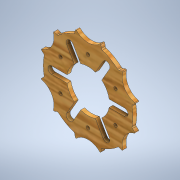
# Autodesk Inventor part: GenevaHolder
Saved by Autodesk Inventor 2020.1 (Build 241239000, 239)
## iProperties
Created: 2019-11-06
Part Number: GenevaHolder
Material: Plywood, Finish
Document SubType Name: Modeling
Designer: Paul Lefeuvre
Density: 0.552 g/cm^3
Appearance: Plywood - New
Author: Paul Lefeuvre
Autodesk Inventor part; units mm, degrees
ref_plane "YZ Plane" through (0, 0, 0) normal (1, 0, 0) x (0, 1, 0)
ref_plane "XZ Plane" through (0, 0, 0) normal (0, 1, 0) x (-1, 0, 0)
ref_plane "XY Plane" through (0, 0, 0) normal (0, 0, 1) x (1, 0, 0)
sketch "Sketch1" plane through (0, 0, 0) normal (0, 0, 1) x (1, 0, 0)
  circle A0 centre (0, 0) radius 175
  circle A1 centre (0, 136.9) radius 38.1
  line L0 (0, 0) -> (0, 152.9684) construction
  circle A2 centre (0, 0) radius 50
  line L1 (0, 0) -> (-42.671, 73.9083)
  line L2 (-31.9973, 38.421) -> (-50.0322, 69.6583)
  line L3 (-17.2749, 46.921) -> (-35.3098, 78.1583)
  arc A3 (-35.3098, 78.1583) -> (-50.0322, 69.6583) centre (-42.671, 73.9083) ccw
  line L4 (-16.7016, 47.1281) -> (-34.7901, 78.4583)
  arc A4 (-34.7901, 78.4583) -> (-50.5518, 69.3583) centre (-42.671, 73.9083) ccw
  line L5 (-50.5518, 69.3583) -> (-32.4633, 38.0281)
  line L6 (-49.1649, 9.1) -> (-85.342, 9.1)
  arc A5 (-85.342, 9.1) -> (-85.342, -9.1) centre (-85.342, 0) ccw
  line L7 (-85.342, -9.1) -> (-49.1649, -9.1)
  line L8 (-49.2722, 8.5) -> (-85.342, 8.5)
  arc A6 (-85.342, 8.5) -> (-85.342, -8.5) centre (-85.342, 0) ccw
  line L9 (-49.2722, -8.5) -> (-85.342, -8.5)
  line L10 (-32.4633, -38.0281) -> (-50.5518, -69.3583)
  arc A7 (-50.5518, -69.3583) -> (-34.7901, -78.4583) centre (-42.671, -73.9083) ccw
  line L11 (-34.7901, -78.4583) -> (-16.7016, -47.1281)
  line L12 (-31.9973, -38.421) -> (-50.0322, -69.6583)
  arc A8 (-50.0322, -69.6583) -> (-35.3098, -78.1583) centre (-42.671, -73.9083) ccw
  line L13 (-17.2749, -46.921) -> (-35.3098, -78.1583)
  line L14 (16.7016, -47.1281) -> (34.7901, -78.4583)
  arc A9 (34.7901, -78.4583) -> (50.5518, -69.3583) centre (42.671, -73.9083) ccw
  line L15 (50.5518, -69.3583) -> (32.4633, -38.0281)
  line L16 (17.2749, -46.921) -> (35.3098, -78.1583)
  arc A10 (35.3098, -78.1583) -> (50.0322, -69.6583) centre (42.671, -73.9083) ccw
  line L17 (31.9973, -38.421) -> (50.0322, -69.6583)
  line L18 (49.1649, -9.1) -> (85.342, -9.1)
  arc A11 (85.342, -9.1) -> (85.342, 9.1) centre (85.342, 0) ccw
  line L19 (85.342, 9.1) -> (49.1649, 9.1)
  line L20 (49.2722, -8.5) -> (85.342, -8.5)
  arc A12 (85.342, -8.5) -> (85.342, 8.5) centre (85.342, 0) ccw
  line L21 (49.2722, 8.5) -> (85.342, 8.5)
  line L22 (32.4633, 38.0281) -> (50.5518, 69.3583)
  arc A13 (50.5518, 69.3583) -> (34.7901, 78.4583) centre (42.671, 73.9083) ccw
  line L23 (34.7901, 78.4583) -> (16.7016, 47.1281)
  line L24 (31.9973, 38.421) -> (50.0322, 69.6583)
  arc A14 (50.0322, 69.6583) -> (35.3098, 78.1583) centre (42.671, 73.9083) ccw
  line L25 (17.2749, 46.921) -> (35.3098, 78.1583)
  arc A15 (49.2722, -8.5) -> (17.2749, 46.921) centre (49.2722, 28.4473) ccw construction
  circle A16 centre (0, 0) radius 93.842 construction
  arc A17 (17.2749, 46.921) -> (49.2722, -8.5) centre (49.2722, 28.4473) ccw construction
  circle A18 centre (49.2722, 28.4473) radius 19.9473 construction
  arc A19 (30.6615, 93.9218) -> (28.3532, 111.45) centre (0, 98.8) ccw
  arc A20 (-28.3532, 111.45) -> (-30.6615, 93.9218) centre (0, 98.8) ccw
  circle A21 centre (0, 0) radius 115 construction
  arc A22 (31.6229, 93.6025) -> (30.2963, 109.2477) centre (0, 98.8) ccw
  arc A23 (-30.2963, 109.2477) -> (-31.6229, 93.6025) centre (0, 98.8) ccw
  arc A24 (-26.9888, 110.0074) -> (26.9888, 110.0074) centre (0, 136.9) ccw
  arc A25 (-26.9888, 110.0074) -> (-30.2963, 109.2477) centre (-28.4056, 108.5957) ccw
  arc A26 (30.2963, 109.2477) -> (26.9888, 110.0074) centre (28.4056, 108.5957) ccw
  arc A27 (31.2727, 102.1077) -> (29.7291, 109.0521) centre (0, 98.8) ccw
  arc A28 (29.7291, 109.0521) -> (27.4139, 109.5839) centre (28.4056, 108.5957) ccw
  arc A29 (-27.4139, 109.5839) -> (27.4139, 109.5839) centre (0, 136.9) ccw
  arc A30 (-27.4139, 109.5839) -> (-29.7291, 109.0521) centre (-28.4056, 108.5957) ccw
  arc A31 (-29.7291, 109.0521) -> (-31.2727, 102.1077) centre (0, 98.8) ccw
  arc A32 (102.8895, -20.9465) -> (102.8895, 20.9465) centre (0, 0) ccw
  arc A33 (-102.8895, 20.9465) -> (-102.8895, -20.9465) centre (0, 0) ccw
  arc A34 (-69.5849, -78.6317) -> (-33.3045, -99.5781) centre (0, 0) ccw
  arc A35 (33.3045, -99.5781) -> (69.5849, -78.6317) centre (0, 0) ccw
  arc A36 (-18.1758, 103.4149) -> (-19.1086, 103.2466) centre (0, 0) ccw
  arc A37 (-33.3045, 99.5781) -> (-69.5849, 78.6317) centre (0, 0) ccw
  arc A38 (69.5849, 78.6317) -> (33.3045, 99.5781) centre (0, 0) ccw
  arc A39 (19.1086, 103.2466) -> (18.1758, 103.4149) centre (0, 0) ccw
  arc A40 (-33.3045, 99.5781) -> (-31.2727, 102.1077) centre (-34.2561, 102.4232) ccw
  arc A41 (31.2727, 102.1077) -> (33.3045, 99.5781) centre (34.2561, 102.4232) ccw
  arc A42 (-102.8895, 20.9465) -> (-104.0642, 23.9709) centre (-105.8292, 21.545) ccw
  arc A43 (-109.3065, 28.7799) -> (-104.0642, 23.9709) centre (-85.5633, 49.4) ccw
  arc A44 (-108.6094, 31.0508) -> (-109.3065, 28.7799) centre (-108.2494, 29.6979) ccw
  arc A45 (-108.6094, 31.0508) -> (-81.1955, 78.533) centre (-118.5589, 68.45) ccw
  arc A46 (-79.5774, 80.2722) -> (-81.1955, 78.533) centre (-79.8439, 78.8978) ccw
  arc A47 (-72.7915, 78.1368) -> (-79.5774, 80.2722) centre (-85.5633, 49.4) ccw
  arc A48 (-72.7915, 78.1368) -> (-69.5849, 78.6317) centre (-71.5731, 80.8783) ccw
  arc A49 (-69.5849, -78.6317) -> (-72.7915, -78.1368) centre (-71.5731, -80.8783) ccw
  arc A50 (-79.5774, -80.2722) -> (-72.7915, -78.1368) centre (-85.5633, -49.4) ccw
  arc A51 (-81.1955, -78.533) -> (-79.5774, -80.2722) centre (-79.8439, -78.8978) ccw
  arc A52 (-81.1955, -78.533) -> (-108.6094, -31.0508) centre (-118.5589, -68.45) ccw
  arc A53 (-109.3065, -28.7799) -> (-108.6094, -31.0508) centre (-108.2494, -29.6979) ccw
  arc A54 (-104.0642, -23.9709) -> (-109.3065, -28.7799) centre (-85.5633, -49.4) ccw
  arc A55 (-104.0642, -23.9709) -> (-102.8895, -20.9465) centre (-105.8292, -21.545) ccw
  arc A56 (33.3045, -99.5781) -> (31.2727, -102.1077) centre (34.2561, -102.4232) ccw
  arc A57 (29.7291, -109.0521) -> (31.2727, -102.1077) centre (0, -98.8) ccw
  arc A58 (27.4139, -109.5839) -> (29.7291, -109.0521) centre (28.4056, -108.5957) ccw
  arc A59 (27.4139, -109.5839) -> (-27.4139, -109.5839) centre (0, -136.9) ccw
  arc A60 (-29.7291, -109.0521) -> (-27.4139, -109.5839) centre (-28.4056, -108.5957) ccw
  arc A61 (-31.2727, -102.1077) -> (-29.7291, -109.0521) centre (0, -98.8) ccw
  arc A62 (-31.2727, -102.1077) -> (-33.3045, -99.5781) centre (-34.2561, -102.4232) ccw
  arc A63 (102.8895, -20.9465) -> (104.0642, -23.9709) centre (105.8292, -21.545) ccw
  arc A64 (109.3065, -28.7799) -> (104.0642, -23.9709) centre (85.5633, -49.4) ccw
  arc A65 (108.6094, -31.0508) -> (109.3065, -28.7799) centre (108.2494, -29.6979) ccw
  arc A66 (108.6094, -31.0508) -> (81.1955, -78.533) centre (118.5589, -68.45) ccw
  arc A67 (79.5774, -80.2722) -> (81.1955, -78.533) centre (79.8439, -78.8978) ccw
  arc A68 (72.7915, -78.1368) -> (79.5774, -80.2722) centre (85.5633, -49.4) ccw
  arc A69 (72.7915, -78.1368) -> (69.5849, -78.6317) centre (71.5731, -80.8783) ccw
  arc A70 (69.5849, 78.6317) -> (72.7915, 78.1368) centre (71.5731, 80.8783) ccw
  arc A71 (79.5774, 80.2722) -> (72.7915, 78.1368) centre (85.5633, 49.4) ccw
  arc A72 (81.1955, 78.533) -> (79.5774, 80.2722) centre (79.8439, 78.8978) ccw
  arc A73 (81.1955, 78.533) -> (108.6094, 31.0508) centre (118.5589, 68.45) ccw
  arc A74 (109.3065, 28.7799) -> (108.6094, 31.0508) centre (108.2494, 29.6979) ccw
  arc A75 (104.0642, 23.9709) -> (109.3065, 28.7799) centre (85.5633, 49.4) ccw
  arc A76 (104.0642, 23.9709) -> (102.8895, 20.9465) centre (105.8292, 21.545) ccw
  arc A77 (-88.2997, 44.3238) -> (-88.2997, -44.3238) centre (0, 0) ccw construction
  arc A78 (-82.5354, -54.3079) -> (-5.7643, -98.6317) centre (0, 0) ccw
  arc A79 (5.7643, -98.6317) -> (82.5354, -54.3079) centre (0, 0) ccw
  arc A80 (88.2997, -44.3238) -> (88.2997, 44.3238) centre (0, 0) ccw
  arc A81 (82.5354, 54.3079) -> (-82.5354, 54.3079) centre (0, 0) ccw
  circle A82 centre (0, 0) radius 74.4
  circle A83 centre (0, 74.4) radius 3.9
  circle A84 centre (-64.4323, 37.2) radius 3.9
  circle A85 centre (-64.4323, -37.2) radius 3.9
  circle A86 centre (0, -74.4) radius 3.9
  circle A87 centre (64.4323, -37.2) radius 3.9
  circle A88 centre (64.4323, 37.2) radius 3.9
  point P0 (-98.9685, 35.0748)
  point P1 (-79.8599, 68.1718)
  point P2 (-79.8599, -68.1718)
  point P3 (-98.9685, -35.0748)
  point P4 (19.1086, -103.2466)
  point P5 (-19.1086, -103.2466)
  point P6 (98.9685, -35.0748)
  point P7 (79.8599, -68.1718)
  point P8 (79.8599, 68.1718)
  point P9 (98.9685, 35.0748)
  point P10 (49.2722, -8.5)
  point P11 (31.9973, -38.421)
  point P12 (17.2749, -46.921)
  point P13 (-17.2749, -46.921)
  point P14 (-31.9973, -38.421)
  point P15 (-49.2722, -8.5)
  point P16 (17.2749, 46.921)
  point P17 (31.9973, 38.421)
  point P18 (49.2722, 8.5)
  dimension "d26" = 148.8
  dimension "d0" = 350
  dimension "d1" = 76.2
  dimension "d2" = 100
  dimension "d3" = 30
  dimension "d4" = 17
  dimension "d5" = 0.6
  dimension "d8" = 360
  dimension "d10" = 230
  dimension "d12" = 1
  dimension "d13" = 1
  dimension "d14" = 2
  dimension "d15" = 0.6
  dimension "d20" = 3
  dimension "d21" = 3
  dimension "d24" = 360
  dimension "d27" = 7.8
  dimension "d30" = 360
  constraints: 192 point on circle, 87 centre point, 52 end point, 16 tangent, 14 coincident, 3 parallel, 2 point on line, 1 equal radius, 1 vertical, 1 vertical alignment, 260 other
  measures "d0" diameter of A0
  measures "d1" diameter of A1
  measures "d2" diameter of A2
  measures "d3" angle of L0 L1
  measures "d4" distance between parallel lines of L2 L3
  measures "d5" distance between parallel lines of L3 L4
  measures "d10" diameter of A21
  measures "d12" radial gap between concentric circles of A19 A22
  measures "d13" radial gap between concentric circles of A20 A23
  measures "d14" radius of A25
  measures "d15" radial gap between concentric circles of A22 A27
  measures "d20" radius of A40
  measures "d21" radius of A41
  measures "d27" diameter of A83
extrude "Extrusion1" add sketch "Sketch1" along normal blind 9 contours A30 A29 A81 A20 | A20 A81 A23 A40 A31 A30 | A28 A27 A41 A22 A81 A19 | A19 A81 A29 A28 | A81 A29 A73 A80 A66 A79 A59 A78 A52 A53 A54 A55 A33 A42 A43 A44 A45 | A23 A81 A45 A46 A47 A48 A37 A40 | A41 A38 A70 A71 A72 A73 A81 A22 | A73 A74 A75 A76 A32 A63 A64 A65 A66 A80 | A66 A67 A68 A69 A35 A56 A57 A58 A59 A79 | A59 A60 A61 A62 A34 A49 A50 A51 A52 A78 | A2 L19 A82 L21 | L20 A82 L18 A2 | A2 L22 A82 A88 L19 | A82 L19 A11 L18 L20 A12 L21 | L18 A82 A87 L15 A2 | A2 L24 A82 L22 | L15 A82 L17 A2 | A82 L24 A14 L25 L23 A13 L22 | L15 A9 L14 A82 L16 A10 L17 | A2 L23 A82 L25 | L16 A82 L14 A2 | A2 L4 A82 A83 L23 | L14 A82 A86 L11 A2 | A2 L3 A82 L4 | L11 A82 L13 A2 | A82 L3 A3 L2 L5 A4 L4 | L11 A7 L10 A82 L12 A8 L13 | L12 A82 L10 A2 | A2 L5 A82 L2 | L10 A82 A85 L7 A2 | A2 L6 A82 A84 L5 | L7 A82 L9 A2 | A2 L8 A82 L6 | L7 A5 L6 A82 L8 A6 L9
body "Solid1"
